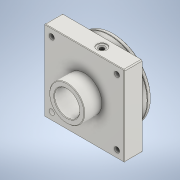
# Autodesk Inventor part: Deckel_vorne
Saved by Autodesk Inventor 2020.3 (Build 243373000, 373)
## iProperties
Created: 2021-05-20
Part Number: Deckel_vorne
Material: Stahl AISI 4130
Document SubType Name: Modeling
Designer: Preuß P. Ch.
Density: 7.85 g/cm^3
Appearance: Stahl
Author: Preuß P. Ch.
Autodesk Inventor part; units mm, degrees
ref_plane "YZ Plane" through (0, 0, 0) normal (1, 0, 0) x (0, 1, 0)
ref_plane "XZ Plane" through (0, 0, 0) normal (0, 1, 0) x (-1, 0, 0)
ref_plane "XY Plane" through (0, 0, 0) normal (0, 0, 1) x (1, 0, 0)
sketch "Skizze1" plane through (0, 0, 0) normal (0, 0, 1) x (1, 0, 0)
  line L0 (0, 0) -> (22.5, 0)
  line L1 (22.5, 0) -> (22.5, 75)
  line L2 (22.5, 75) -> (0, 75)
  line L3 (0, 75) -> (0, 0)
  line L4 (22.5, 80) -> (57.5, 80)
  line L5 (57.5, 80) -> (57.5, -80)
  line L6 (57.5, -80) -> (22.5, -80)
  line L7 (22.5, -80) -> (22.5, 80)
  line L8 (57.5, 0) -> (92.5, 0)
  line L9 (92.5, 0) -> (92.5, 35)
  line L10 (92.5, 35) -> (57.5, 35)
  line L11 (57.5, 35) -> (57.5, 0)
  line L12 (6, 75) -> (7.5, 75)
  line L13 (7.5, 75) -> (7.5, 73.5)
  line L14 (7.5, 73.5) -> (6, 73.5)
  line L15 (6, 73.5) -> (6, 75)
  dimension "d9" = 160
  dimension "d10" = 70
  dimension "d11" = 150
  dimension "d12" = 22.5
  dimension "d13" = 35
  dimension "d14" = 92.5
  dimension "d15" = 6
  dimension "d16" = 1.5
  dimension "d17" = 147
  constraints: 32 end point, 8 parallel, 4 horizontal, 4 perpendicular, 2 midpoint, 2 point on line
  measures "d9" diameter of L4 L0
  measures "d10" diameter of L10 L0
  measures "d11" diameter of L2 L0
  measures "d12" distance between parallel lines of L1 L3
  measures "d13" distance between parallel lines of L5 L1
  measures "d14" distance between parallel lines of L9 L3
  measures "d15" distance between parallel lines of L15 L3
  measures "d16" distance between parallel lines of L13 L15
  measures "d17" diameter of L14 L0
revolve "Umdrehung1" add sketch "Skizze1" angle 360 about axis through (0, 0, 0) along (1, 0, 0) contours L3 L2 L15 L14 L13 L1 L0 | L5 L10 L9 L8
extrude "Extrusion1" add sketch "Skizze1" along normal mid plane 160 contours L1 L7 L4 L5 L6
sketch "Skizze2" plane through (92.5, 0, 0) normal (1, 0, 0) x (0, 0, -1)
  circle A0 centre (0, 0) radius 35 projected
  constraints: 1 coincident
hole "Bohrung1" at (92.5, 0, 0) direction (-1, 0, 0) diameter 50 end through all
sketch "Skizze3" plane through (57.5, -80, 80) normal (1, 0, 0) x (0, 0, -1)
  line L0 (0, 160) -> (160, 160) projected
  line L1 (0, 160) -> (30, 160)
  line L2 (30, 160) -> (30, 130)
  line L3 (30, 130) -> (0, 130)
  line L4 (0, 130) -> (0, 160)
  line L5 (145, 15) -> (15, 15)
  line L6 (15, 15) -> (15, 145)
  line L7 (15, 145) -> (145, 145)
  line L8 (145, 145) -> (145, 15)
  line L9 (145, 15) -> (15, 145) construction
  line L10 (15, 15) -> (145, 145) construction
  point P0 (80, 80)
  dimension "d28" = 30
  dimension "d29" = 30
  dimension "d30" = 130
  dimension "d31" = 130
  constraints: 20 end point, 4 parallel, 2 horizontal, 2 midpoint, 2 perpendicular
  measures "d28" distance of L2.end L3.end
  measures "d29" distance of L1.end L2.end
  measures "d30" distance of L6.end L7.end
  measures "d31" distance of L5.end L6.end
hole "Bohrung2" at (57.5, 65, 65) direction (-1, 0, 0) diameter 10.5 end through all
pattern_circular "Runde Anordnung1" count 4 over 360 about axis through (75, 0, 0) along (1, 0, 0) of "Bohrung2"
sketch "Skizze5" plane through (0, 0, 0) normal (-1, 0, 0) x (0, 0, 1)
  line L0 (80, 80) -> (-80, 80) projected
  line L1 (-80, 80) -> (-80, -80) projected
  point P0 (0, 0)
  point P1 (-17.5, 50)
  point P2 (-80, 50)
  point P3 (-80, -50)
  dimension "d54" = 30
  dimension "d55" = 62.5
  measures "d54" distance from line of L0 point (-17.5, 50)
  measures "d55" distance from line of L1 point (-17.5, 50)
hole "Bohrung3" at (0, 50, -17.5) direction (1, 0, 0) diameter 8.5 depth 36 tip angle 118
sketch "Skizze6" plane through (22.5, 80, 80) normal (0, 1, 0) x (1, 0, 0)
  line L0 (35, 160) -> (35, 0) projected
  line L1 (5, 160) -> (35, 160) projected
  point P0 (-22.5, 80)
  point P1 (17.5, 97.5)
  point P2 (35, 130)
  point P3 (35, 30)
  dimension "d63" = 17.5
  dimension "d64" = 62.5
  measures "d63" distance from line of L0 point (17.5, 97.5)
  measures "d64" distance from line of L1 point (17.5, 97.5)
hole "Bohrung4" at (40, 80, -17.5) direction (0, -1, 0) diameter 8.376 depth 34.5 tip angle 118 counterbore diameter 20 counterbore depth 1.5 thread size "M10x1.5" class "6H" standard "ISO Metric profile"
chamfer "Fase1" distance 2 angle 45 1 edges at (40, 78.5, -21.688)
chamfer "Fase2" distance 1 angle 45 8 edges at (0, -75, 0) (0, 0, 25) (92.5, 0, 25) (92.5, -35, 0) (57.5, 0, 80) (57.5, 80, 0) (57.5, 0, -80) (57.5, -80, 0)
fillet "Rundung2" radius 2 4 edges at (39.5, 80, -80) (39.5, 80, 80) (39.5, -80, -80) (39.5, -80, 80)
equation "\"d19\" = d9"
